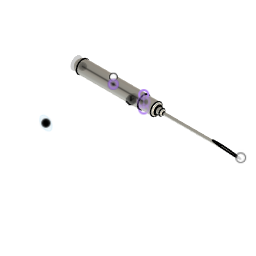
Link_EF (Autodesk Fusion 360 design; units mm, degrees)
Autodesk Fusion 360 part; units mm, degrees
sketch "Boceto1" plane through (0, 0, 0) normal (1, 0, 0) x (0, 0, -1)
  circle A0 centre (0, 0) radius 25
  dimension "d1" = 50
  constraint coincident A0.centre origin
  measures "d1" diameter of A0
extrude "Extruir1" add sketch "Boceto1" along normal blind 270
fillet "Empalme1" radius 25 1 edges at (0, -9.0404, 23.3082)
sketch "Boceto2" plane through (270, 0, 0) normal (1, 0, 0) x (0, 0, -1)
  circle A0 centre (0, 0) radius 25
  circle A1 centre (0, 0) radius 5
  circle A2 centre (0, 0) radius 3.75
  dimension "d6" = 10
  dimension "d9" = 7.5
  constraint concentric A0 A1
  constraint concentric A1 A2
  measures "d6" diameter of A1
  measures "d9" diameter of A2
extrude "Extruir3" add sketch "Boceto2" along normal blind 400 contours A1
ref_plane "PlanoDeObra1" through (0, 12.125, 0) normal (0.996195, 0, -0.087156) x (0, 1, 0)
sketch "Boceto3" plane through (0, 0, 0) normal (0.996195, 0, -0.087156) x (0, 1, 0)
  line L0 (7.3769, 52.429) -> (-7.4393, 52.429)
  line L1 (-7.4393, 52.429) -> (-7.4393, 64.619)
  line L2 (-7.4393, 64.619) -> (7.3769, 64.619)
  line L3 (7.3769, 64.619) -> (7.3769, 52.429)
  line L4 (7.3769, 52.429) -> (-7.4393, 64.619) construction
  line L5 (-7.4393, 52.429) -> (7.3769, 64.619) construction
  constraint horizontal L0
  constraint perpendicular L0 L1
  constraint parallel L0 L2
  constraint parallel L1 L3
extrude "Extruir4" cut sketch "Boceto3" along normal blind 750
sketch "Boceto5" plane through (0, 0, 0) normal (0, 0, 1) x (1, 0, 0)
  line L0 (270, 0) -> (327.5939, 0)
  line L1 (327.5939, 0) -> (327.5939, -23.2586)
  line L2 (327.5939, -23.2586) -> (270, -23.2586)
  line L3 (270, -23.2586) -> (270, 0)
  line L4 (327.5939, 0) -> (350.0814, 0)
  line L5 (350.0814, 0) -> (350.0814, -11.6293)
  line L6 (350.0814, -11.6293) -> (327.5939, -11.6293)
  line L7 (327.5939, -11.6293) -> (327.5939, 0)
  constraint horizontal L0
  constraint vertical L1
  constraint horizontal L2
  constraint vertical L3
  constraint horizontal L4
  constraint vertical L5
  constraint horizontal L6
  constraint vertical L7
revolve "Revolución1" add sketch "Boceto5" angle 360 about axis through (327.5939, 0, 0) along (1, 0, 0)
fillet "Empalme2" radius 7.5 2 edges at (350.0814, -4.2053, -10.8423) (327.5939, -8.4107, -21.6846)
move_body "Desplazar1" bodies 1 to x (0, 0, 1) y (0, 1, 0) z (-1, 0, 0) at (342.6321, 0, -342.6321)
move_body "Desplazar2" bodies 1 to x (0, 0.017452, -0.999848) y (0, 0.999848, 0.017452) z (1, 0, 0) at (335.1828, -5.9798, 350.0292)
move_body "Desplazar3" bodies 1 to x (0, 0.999848, 0.017452) y (-0.999848, 0.000305, -0.01745) z (-0.017452, -0.01745, 0.999695) at (312.7746, -312.467, -5.4541)
move_body "Desplazar4" bodies 1 to x (1, 0, 0) y (0, 1, 0) z (0, 0, 1) at (-600, 5.2357, -299.9543)
move_body "Desplazar5" bodies 1 to x (1, 0, 0) y (0, 1, 0) z (0, 0, 1) at (300, -5.2357, 299.9543)
move_body "Desplazar6" bodies 1 to x (1, 0, 0) y (0, 1, 0) z (0, 0, 1) at (-3.4586, -6.6612, -19.4692)
move_body "Desplazar7" bodies 1 to x (1, 0, 0) y (0, 1, 0) z (0, 0, 1) at (0, 56.5914, 0.9878)
move_body "Move8" bodies 1 to x (1, 0, 0) y (0, 0.999848, -0.017452) z (0, 0.017452, 0.999848) at (0, 0.1967, 1.2631)
sketch "Sketch6" plane through (0, 79.9142, 0) normal (0, 1, 0) x (-1, 0, 0)
  circle A0 centre (-9.186, -10.6388) radius 3.75
  line L0 (-9.186, -10.6388) -> (-9.186, 0)
  line L1 (-9.186, 0) -> (-9.186, -10.6388)
  line L2 (-9.186, -10.6388) -> (0, -10.6388)
  dimension "d18" = 10.6388
  dimension "d19" = 9.186
  constraint coincident A0.centre L0.start
  constraint vertical L0
  constraint perpendicular L0 L2
  measures "d18" distance of A0.centre L0.end
  measures "d19" distance of A0.centre L2.end
move_body "Move10" bodies 1 to x (1, 0, 0) y (0, 1, 0) z (0, 0, 1) at (-9.186, 122.2872, 10.5985)
sketch "Sketch7" plane through (0, 0, 0) normal (1, 0, 0) x (0, 1, 0)
  line L0 (0.76, 24.96) -> (0, 24.96)
  line L1 (0, 0) -> (-122.88, 0)
  line L2 (0, 0) -> (122.12, 0)
  dimension "d22" = 122.88
  dimension "d23" = 122.12
  constraint horizontal L0
  constraint coincident L1.start L2.start
  constraint horizontal L1
  constraint parallel L1 L2
  measures "d22" distance of L1.end L1.start
  measures "d23" distance of L2.end L1.start
sketch "Sketch8" plane through (0, 0, 0) normal (1, 0, 0) x (0, 1, 0)
  line L0 (122.1201, -25.0403) -> (122.1201, 24.9597)
  dimension "d24" = 122.1201
  measures "d24" distance of origin L0
sketch "Sketch9" plane through (0, 0, 0) normal (0, 0, 1) x (1, 0, 0)
  point P0 (0, 510.825)
  point P1 (0, 122.12)
  dimension "d25" = 388.705
  measures "d25" distance of P0 P1
